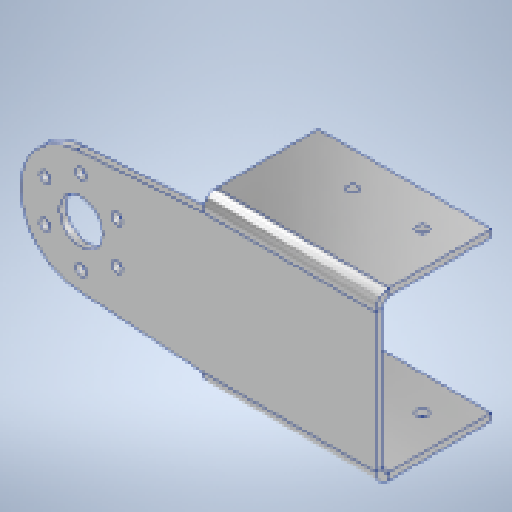
# Autodesk Inventor part: servoplate1_forR2
Saved by Autodesk Inventor 2024.3 (Build 283343010, 343A)
## iProperties
Created: 2025-05-29
Part Number: servoplate1_forR2
Material: アルミニウム 6061
Document SubType Name: Sheet Metal
Designer: kshau
Density: 2.7 g/cm^3
Sheet Metal Rule: Default
Appearance: アルミニウム - フラット
Author: kshau
Autodesk Inventor part; units mm, degrees
ref_plane "YZ Plane" through (0, 0, 0) normal (1, 0, 0) x (0, 1, 0)
ref_plane "XZ Plane" through (0, 0, 0) normal (0, 1, 0) x (-1, 0, 0)
ref_plane "XY Plane" through (0, 0, 0) normal (0, 0, 1) x (1, 0, 0)
sketch "スケッチ1" plane through (0, 0, 0) normal (0, 0, 1) x (1, 0, 0)
  circle A0 centre (0, 0) radius 17.5
  line L0 (0, 0) -> (35, 0)
  line L1 (35, 0) -> (35, 20)
  line L2 (35, 20) -> (-1.2255, 17.457)
  line L3 (35, 20) -> (85, 20)
  line L4 (85, 20) -> (85, 0)
  line L5 (85, 0) -> (35, 0)
  line L6 (35, 0) -> (35, 20)
  line L7 (35, 0) -> (35, -20)
  line L8 (35, -20) -> (-1.2255, -17.457)
  line L9 (35, -20) -> (85, -20)
  line L10 (85, -20) -> (85, 0)
  point P0 (-1.2255, -17.457)
  dimension "d0" = 35
  dimension "d1" = 35
  dimension "d2" = 20
  dimension "d3" = 20
  dimension "d4" = 50
  measures "d1" distance of L0.start L0.end
  measures "d2" distance of L0.end L1.end
  measures "d3" distance of L3.end L4.end
  measures "d4" distance of L4.end L5.end
extrude "プレート1" add sketch "スケッチ1" along normal blind 2
sketch "スケッチ2" plane through (85, 22, -2) normal (0, 1, 0) x (-1, 0, 0)
  line L0 (50, 0) -> (0, 0)
  line L1 (0, 0) -> (0, -29.5)
  line L2 (0, -29.5) -> (50, -29.5)
  line L3 (50, -29.5) -> (50, 0)
  constraints: 6 end point, 1 horizontal, 1 perpendicular, 1 vertical
edge flange "フランジ1" height 33.5 angle 90 thickness 2 bend radius 2 thickness toward (0, 1, 0) relief straight relief width 2 relief depth 1 corner gap 2 corner form 0 edges at (60, 20, 0) (60, -20, 0) wall of the first edge with corners at (35, 22, -2) (85, 22, -2) (85, 22, -31.5) (35, 22, -31.5)
bend "曲げ1"
corner "コーナー1"
sketch "スケッチ3" plane through (0, 0, 2) normal (0, 0, 1) x (1, 0, 0)
  circle A0 centre (0, 0) radius 13.5
  point P0 (0, 13.5)
  point P1 (-11.6913, 6.75)
  point P2 (-11.6913, -6.75)
  point P3 (0, -13.5)
  point P4 (11.6913, -6.75)
  point P5 (11.6913, 6.75)
  dimension "d16" = 27
  dimension "d19" = 360
  constraints: 1 coincident, 1 vertical alignment, 9 other
hole "穴1" at (0, 13.5, 2) at (-11.6913, 6.75, 2) at (-11.6913, -6.75, 2) at (0, -13.5, 2) at (11.6913, -6.75, 2) at (11.6913, 6.75, 2) direction (0, 0, -1) diameter 3.2 end through all
sketch "スケッチ4" plane through (0, 0, 2) normal (0, 0, 1) x (1, 0, 0)
  arc A0 (-1.2255, 17.457) -> (-1.2255, -17.457) centre (0, 0) ccw projected
  circle A1 centre (0, 0) radius 6.25
  dimension "d28" = 12.5
  constraints: 1 centre point, 1 coincident
  measures "d28" diameter of A1
extrude "押し出し1" cut sketch "スケッチ4" against normal blind 10
sketch "スケッチ5" plane through (35, 24, -31.5) normal (0, 1, 0) x (1, 0, 0)
  line L0 (0, 0) -> (0, -29.5) projected
  line L1 (0, -10) -> (50, -10)
  line L2 (50, -29.5) -> (50, 0) projected
  line L3 (50, 0) -> (0, 0) projected
  line L4 (10, 0) -> (10, -29.5)
  line L5 (0, -29.5) -> (50, -29.5) projected
  point P0 (-35, -31.5)
  point P1 (20, -10)
  point P2 (40, -10)
  dimension "d31" = 10
  dimension "d32" = 10
  dimension "d33" = 10
  dimension "d34" = 20
  constraints: 6 point on line, 4 end point, 1 horizontal, 1 perpendicular
  measures "d31" distance between parallel lines of L0 L4
  measures "d32" distance between parallel lines of L3 L1
  measures "d33" distance from line of L4 point (20, -10)
  measures "d34" distance of point (20, -10) point (40, -10)
hole "穴2" at (55, 24, -21.5) at (75, 24, -21.5) direction (0, -1, 0) diameter 3.2 end through all
equation "\"d26\" = Thickness"
equation "\"d5\" = Thickness"
equation "\"d6\" = BendReliefWidth"
equation "\"d7\" = BendReliefDepth"
equation "\"d8\" = MinimumRemnant"
equation "\"d9\" = TransitionRadius"
equation "\"d12\" = BendRadius"
equation "\"d13\" = CornerReliefSize"
equation "\"d14\" = GapSize"
equation "\"d15\" = JacobiRadiusSize"
equation "\"BendRadius\" = Thickness"
equation "\"BendReliefWidth\" = Thickness"
equation "\"BendReliefDepth\" = 0.5 * Thickness"
equation "\"CornerReliefSize\" = 4 * Thickness"
equation "\"MinimumRemnant\" = 2 * Thickness"
equation "\"TransitionRadius\" = BendRadius"
equation "\"JacobiRadiusSize\" = BendRadius"
equation "\"GapSize\" = Thickness"
equation "\"Thickness\" = 2"
